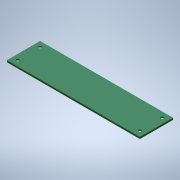
# Autodesk Inventor part: tapa
Saved by Autodesk Inventor 2021 (Build 250183000, 183)
## iProperties
Created: 2021-03-08
Part Number: tapa
Material: Steel, Mild, Welded
Document SubType Name: Modeling
Designer: Usuario
Density: 7.85 g/cm^3
Appearance: Smooth - Dark Sea Green
Author: Usuario
Autodesk Inventor part; units mm, degrees
ref_plane "YZ Plane" through (0, 0, 0) normal (1, 0, 0) x (0, 1, 0)
ref_plane "XZ Plane" through (0, 0, 0) normal (0, 1, 0) x (-1, 0, 0)
ref_plane "XY Plane" through (0, 0, 0) normal (0, 0, 1) x (1, 0, 0)
sketch "Sketch1" plane through (0, 0, 0) normal (0, 1, 0) x (-1, 0, 0)
  line L0 (76, 19) -> (-76, 19)
  line L1 (-76, 19) -> (-76, -19)
  line L2 (-76, -19) -> (76, -19)
  line L3 (76, -19) -> (76, 19)
  line L4 (76, 19) -> (-76, -19) construction
  line L5 (-76, 19) -> (76, -19) construction
  point P0 (0, 0)
  dimension "d0" = 152
  dimension "d1" = 38
  constraints: 12 end point, 2 midpoint, 2 parallel, 1 horizontal, 1 perpendicular
  measures "d0" distance of L2.end L1.end
  measures "d1" distance of L1.end L0.end
extrude "Extrusion1" add sketch "Sketch1" along normal blind 2
sketch "Sketch2" plane through (0, 0, 0) normal (0, -1, 0) x (1, 0, 0)
  line L0 (76, 19) -> (76, -19) projected
  line L1 (-76, 19) -> (76, 19) projected
  line L2 (-76, -19) -> (-76, 19) projected
  line L3 (76, -19) -> (-76, -19) projected
  line L4 (-76, -19) -> (-76, 19) projected
  line L5 (-76, 19) -> (76, 19) projected
  line L6 (-76, -19) -> (76, -19)
  line L7 (76, -19) -> (76, 19)
  line L8 (76, 19) -> (-76, 19)
  line L9 (-76, 19) -> (-76, -19)
  line L10 (-76, -19) -> (-75.15, -19)
  line L11 (76, -19) -> (-76, -19) projected
  line L12 (76, 19) -> (76, 18.15)
  line L13 (76, 19) -> (76, -19) projected
  line L14 (-74.85, -18.35) -> (74.85, -18.35)
  line L15 (75.35, -17.85) -> (75.35, 17.85)
  line L16 (74.85, 18.35) -> (-74.85, 18.35)
  line L17 (-75.35, 17.85) -> (-75.35, -17.85)
  line L18 (75.35, -18.35) -> (74.4, -18.35)
  line L19 (-75.35, 18.35) -> (-74.4, 18.35)
  line L20 (73.35, -16.85) -> (-73.35, -16.85)
  line L21 (-73.85, -16.35) -> (-73.85, 16.35)
  line L22 (-73.35, 16.85) -> (73.35, 16.85)
  line L23 (73.85, 16.35) -> (73.85, -16.35)
  arc A0 (-74.85, 18.35) -> (-75.35, 17.85) centre (-74.85, 17.85) ccw
  arc A1 (-73.35, 16.85) -> (-73.85, 16.35) centre (-73.35, 16.35) ccw
  arc A2 (-75.35, -17.85) -> (-74.85, -18.35) centre (-74.85, -17.85) ccw
  arc A3 (-73.85, -16.35) -> (-73.35, -16.85) centre (-73.35, -16.35) ccw
  arc A4 (73.35, -16.85) -> (73.85, -16.35) centre (73.35, -16.35) ccw
  arc A5 (74.85, -18.35) -> (75.35, -17.85) centre (74.85, -17.85) ccw
  arc A6 (73.85, 16.35) -> (73.35, 16.85) centre (73.35, 16.35) ccw
  arc A7 (75.35, 17.85) -> (74.85, 18.35) centre (74.85, 17.85) ccw
  point P0 (0, 0)
  point P1 (-75.35, -18.35)
  point P2 (75.35, 18.35)
  point P3 (73.85, -16.85)
  point P4 (-73.85, 16.85)
  point P5 (-73.85, -16.85)
  point P6 (73.85, 16.85)
  dimension "d28" = 1.5
  dimension "d29" = 1.5
  dimension "d30" = 1.5
  dimension "d32" = 1.5
  dimension "d33" = 0.65
  dimension "d34" = 0.65
  dimension "d35" = 0.65
  dimension "d36" = 0.65
  dimension "d37" = 0.5
  constraints: 32 end point, 20 point on line, 16 point on circle, 16 tangent, 8 centre point, 7 equal radius, 6 parallel, 3 horizontal, 3 perpendicular
  measures "d28" distance between parallel lines of L21 L17
  measures "d29" distance between parallel lines of L22 L16
  measures "d30" distance between parallel lines of L20 L14
  measures "d32" distance between parallel lines of L23 L15
  measures "d33" distance between parallel lines of L15 L0
  measures "d34" distance between parallel lines of L16 L1
  measures "d35" distance between parallel lines of L14 L3
  measures "d36" distance between parallel lines of L2 L17
  measures "d37" radius of A0
extrude "Extrusion2" cut sketch "Sketch2" against normal blind 0.75 contours A2 L17 A0 L16 A7 L15 A5 L14 | L20 A3 L21 A1 L22 A6 L23 A4
sketch "Sketch3" plane through (0, 0, 0) normal (0, -1, 0) x (1, 0, 0)
  line L0 (-74.85, 18.35) -> (74.85, 18.35) projected
  line L1 (-75.35, -17.85) -> (-75.35, 17.85) projected
  line L2 (74.85, -18.35) -> (-74.85, -18.35) projected
  line L3 (75.35, 17.85) -> (75.35, -17.85) projected
  line L4 (76, 19) -> (76, -19) projected
  line L5 (-76, 19) -> (76, 19) projected
  line L6 (-76, -19) -> (-76, 19) projected
  line L7 (76, -19) -> (-76, -19) projected
  line L8 (-75.35, -17.85) -> (-75.35, 17.85) projected
  line L9 (-74.85, 18.35) -> (74.85, 18.35) projected
  line L10 (75.35, 17.85) -> (75.35, -17.85) projected
  line L11 (74.85, -18.35) -> (-74.85, -18.35) projected
  line L12 (-73.85, 16.85) -> (-73.85, -16.85) projected
  line L13 (-73.85, -16.85) -> (73.85, -16.85) projected
  line L14 (73.85, -16.85) -> (73.85, 16.85) projected
  line L15 (73.85, 16.85) -> (-73.85, 16.85) projected
  line L16 (-73.85, 16.85) -> (-73.85, -16.85) projected
  line L17 (-73.85, 16.85) -> (-65.85, 16.85)
  line L18 (-65.85, 16.85) -> (-65.85, 8.85)
  line L19 (-65.85, 8.85) -> (-73.85, 8.85)
  line L20 (-73.85, 8.85) -> (-73.85, 16.85)
  line L21 (-73.85, -16.85) -> (-65.85, -16.85)
  line L22 (-65.85, -16.85) -> (-65.85, -8.85)
  line L23 (-65.85, -8.85) -> (-73.85, -8.85)
  line L24 (-73.85, -8.85) -> (-73.85, -16.85)
  line L25 (73.85, -16.85) -> (73.85, 16.85) projected
  line L26 (73.85, 16.85) -> (65.85, 16.85)
  line L27 (65.85, 16.85) -> (65.85, 8.85)
  line L28 (65.85, 8.85) -> (73.85, 8.85)
  line L29 (73.85, 8.85) -> (73.85, 16.85)
  line L30 (-73.85, -16.85) -> (73.85, -16.85) projected
  line L31 (73.85, -16.85) -> (65.85, -16.85)
  line L32 (65.85, -16.85) -> (65.85, -8.85)
  line L33 (65.85, -8.85) -> (73.85, -8.85)
  line L34 (73.85, -8.85) -> (73.85, -16.85)
  line L35 (-73.85, -16.85) -> (-65.85, -8.85)
  line L36 (-65.85, -16.85) -> (-73.85, -8.85)
  line L37 (-73.85, 8.85) -> (-65.85, 16.85)
  line L38 (73.85, 16.85) -> (-73.85, 16.85) projected
  line L39 (-65.85, 8.85) -> (-73.85, 16.85)
  circle A0 centre (-69.85, -12.85) radius 1.65
  circle A1 centre (-69.85, 12.85) radius 1.65
  line L40 (65.85, -16.85) -> (73.85, -8.85)
  line L41 (65.85, 8.85) -> (73.85, 16.85)
  line L42 (73.85, 8.85) -> (65.85, 16.85)
  line L43 (73.85, -16.85) -> (65.85, -8.85)
  circle A2 centre (69.85, -12.85) radius 1.65
  circle A3 centre (69.85, 12.85) radius 1.65
  arc A4 (-75.35, -17.85) -> (-74.85, -18.35) centre (-74.85, -17.85) ccw projected
  arc A5 (-74.85, 18.35) -> (-75.35, 17.85) centre (-74.85, 17.85) ccw projected
  arc A6 (75.35, 17.85) -> (74.85, 18.35) centre (74.85, 17.85) ccw projected
  arc A7 (74.85, -18.35) -> (75.35, -17.85) centre (74.85, -17.85) ccw projected
  arc A8 (-75.35, -17.85) -> (-74.85, -18.35) centre (-74.85, -17.85) ccw projected
  arc A9 (74.85, -18.35) -> (75.35, -17.85) centre (74.85, -17.85) ccw projected
  arc A10 (75.35, 17.85) -> (74.85, 18.35) centre (74.85, 17.85) ccw projected
  arc A11 (-74.85, 18.35) -> (-75.35, 17.85) centre (-74.85, 17.85) ccw projected
  point P0 (0, 0)
  dimension "d14" = 8
  dimension "d15" = 8
  dimension "d16" = 8
  dimension "d17" = 8
  dimension "d18" = 8
  dimension "d19" = 8
  dimension "d20" = 8
  dimension "d21" = 8
  dimension "d22" = 3.3
  dimension "d23" = 3.3
  dimension "d24" = 3.3
  dimension "d25" = 3.3
  constraints: 48 end point, 8 parallel, 4 centre point, 4 horizontal, 4 midpoint, 4 perpendicular
  measures "d14" distance of L18.end L19.end
  measures "d15" distance of L17.end L18.end
  measures "d16" distance of L23.end L22.end
  measures "d17" distance of L22.end L21.end
  measures "d18" distance of L28.end L27.end
  measures "d19" distance of L27.end L26.end
  measures "d20" distance of L32.end L33.end
  measures "d21" distance of L31.end L32.end
  measures "d22" diameter of A0
  measures "d23" diameter of A1
  measures "d24" diameter of A2
  measures "d25" diameter of A3
extrude "Extrusion3" cut sketch "Sketch3" against normal blind 3 contours A1 L37 L39 | L39 L37 A1 | L37 L39 A1 | A1 L39 L37 | A0 L35 L36 | L36 L35 A0 | A3 L41 L42 | L42 L41 A3 | L35 L36 A0 | A0 L36 L35 | A3 L42 L41 | L41 L42 A3 | A2 L43 L40 | L40 L43 A2 | A2 L43 L40 | L40 L43 A2
sketch "Sketch4" plane through (0, 0, 0) normal (0, -1, 0) x (1, 0, 0)
  point P0 (0, 0)
body "Solid1"
